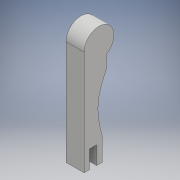
# Autodesk Inventor part: Puente
Saved by Autodesk Inventor 2017 SP1 (Build 210196100, 196)
## iProperties
Part Number: Puente
Material: Genérico
Document SubType Name: Modeling
Designer: Juan
Density: 1 g/cm^3
Appearance: Valor por defecto
Author: Juan
Autodesk Inventor part; units mm, degrees
ref_plane "YZ Plane" through (0, 0, 0) normal (1, 0, 0) x (0, 1, 0)
ref_plane "XZ Plane" through (0, 0, 0) normal (0, 1, 0) x (-1, 0, 0)
ref_plane "XY Plane" through (0, 0, 0) normal (0, 0, 1) x (1, 0, 0)
sketch "Boceto1" plane through (0, 0, 0) normal (1, 0, 0) x (0, 1, 0)
  line L0 (10, 13) -> (10, 0)
  line L1 (10, 0) -> (7, 0)
  line L2 (0, 0) -> (3, 0)
  line L3 (0, 13) -> (0, 0)
  line L4 (7, 0) -> (7, 10)
  line L5 (7, 10) -> (3, 10)
  line L6 (3, 10) -> (3, 0)
  line L7 (10, 13) -> (6.6085, 25.8376) construction
  line L8 (6.6085, 25.8376) -> (6.6085, 31.8916) construction
  line L9 (6.6085, 31.8916) -> (12.4332, 43.8228) construction
  spline S0 degree 3 poles (10, 13) (6.6085, 25.8376) (6.6085, 31.8916) (12.4332, 43.8228) knots 1 1 1 1 2 2 2 2
  line L10 (0, 13) -> (0, 58)
  line L11 (12.4332, 43.8228) -> (12.4332, 50.8228)
  arc A0 (12.4332, 50.8228) -> (0, 58) centre (8.2882, 58) ccw
  dimension "d4" = 3
  dimension "d5" = 13
  dimension "d6" = 45
  dimension "d7" = 7
  dimension "d8" = 4
  dimension "d9" = 3
  dimension "d10" = 13
  dimension "d11" = 8.2882
  dimension "d12" = 153.979
  dimension "d13" = 14.799
  dimension "d14" = 2.4332
  dimension "d15" = 5.8247
  dimension "d16" = 10
  constraints: 18 end point, 5 vertical, 2 parallel, 2 point on circle, 2 point on line, 1 centre point, 1 coincident, 1 horizontal, 1 perpendicular, 1 tangent, 3 other
  measures "d4" distance of L2.start L2.end
  measures "d5" distance of L0.start L0.end
  measures "d6" distance of L3.start L10.end
  measures "d7" distance of L9.end L11.end
  measures "d8" distance of L4.end L5.end
  measures "d9" distance of L0.end L1.end
  measures "d10" distance of L3.start L2.start
  measures "d11" radius of A0
  measures "d12" angle of L9 L11
  measures "d13" angle of L7 L11
  measures "d14" distance between parallel lines of L0 L11
  measures "d15" distance between parallel lines of L8 L11
  measures "d16" distance between parallel lines of L5 L1
extrude "Extrusión1" add sketch "Boceto1" along normal blind 10
